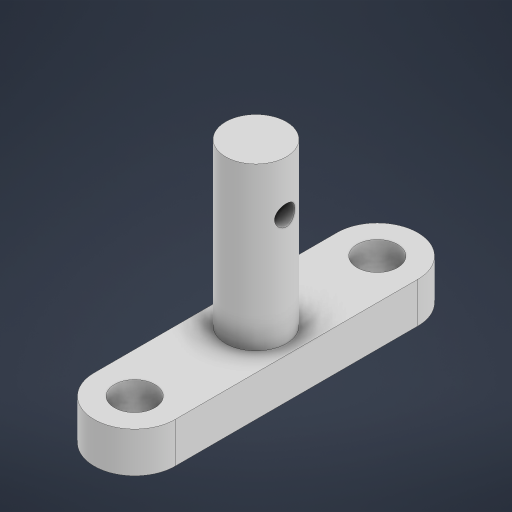
# Autodesk Inventor part: Crank
Saved by Autodesk Inventor 2023.2 (Build 272271000, 271)
## iProperties
Created: 2023-01-16
Part Number: Crank
Material: Generic
Document SubType Name: Modeling
Designer: iusti
Density: 1 g/cm^3
Appearance: Default
Author: iusti
Autodesk Inventor part; units mm, degrees
ref_plane "YZ Plane" through (0, 0, 0) normal (1, 0, 0) x (0, 1, 0)
ref_plane "XZ Plane" through (0, 0, 0) normal (0, 1, 0) x (-1, 0, 0)
ref_plane "XY Plane" through (0, 0, 0) normal (0, 0, 1) x (1, 0, 0)
sketch "Sketch1" plane through (0, 0, 0) normal (0, 1, 0) x (-1, 0, 0)
  line L0 (0, 12) -> (0, -12) construction
  line L1 (-4, 12) -> (-4, -12)
  line L2 (4, -12) -> (4, 12)
  arc A0 (4, 12) -> (-4, 12) centre (0, 12) ccw
  arc A1 (-4, -12) -> (4, -12) centre (0, -12) ccw
  point P0 (0, 0)
  point P1 (0, 0)
  dimension "d0" = 24
  dimension "d1" = 8
  constraints: 8 end point, 4 point on circle, 4 tangent, 2 centre point, 1 coincident, 1 midpoint, 1 parallel, 1 vertical
  measures "d0" distance of L0.start L0.end
  measures "d1" diameter of A1
extrude "Extrusion1" add sketch "Sketch1" along normal blind 4
sketch "Sketch2" plane through (0, 4, 0) normal (0, 1, 0) x (1, 0, 0)
  circle A0 centre (0, 0) radius 3
  dimension "d4" = 6
  constraints: 1 centre point, 1 coincident
  measures "d4" diameter of A0
extrude "Extrusion2" add sketch "Sketch2" along normal blind 16
sketch "Sketch3" plane through (0, 0, 0) normal (1, 0, 0) x (0, 1, 0)
  circle A0 centre (15, 0) radius 1
  line L0 (20, -3) -> (20, 3) projected
  point P0 (0, 0)
  dimension "d7" = 2
  dimension "d8" = 5
  constraints: 1 centre point
  measures "d7" diameter of A0
  measures "d8" distance from line of L0 A0.centre
extrude "Extrusion3" cut sketch "Sketch3" along normal mid plane 16
sketch "Sketch4" plane through (0, 4, 0) normal (0, 1, 0) x (1, 0, 0)
  arc A0 (4, 12) -> (-4, 12) centre (0, 12) ccw projected
  arc A1 (-4, -12) -> (4, -12) centre (0, -12) ccw projected
  constraints: 2 coincident
hole "Hole1" at (0, 4, 12) at (0, 4, -12) direction (0, -1, 0) diameter 4 end through all
body "Solid1"
